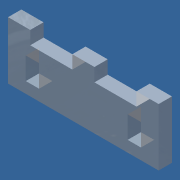
# Autodesk Inventor part: link2p1press
Saved by Autodesk Inventor 2014 (Build 180170000, 170)
## iProperties
Created: 2013-09-11
Part Number: link2p1press
Material: Glass
Document SubType Name: Modeling
Designer: Lefo
Density: 2.18 g/cm^3
Appearance: Clear
Author: Lefo
Autodesk Inventor part; units mm, degrees
ref_plane "YZ Plane" through (0, 0, 0) normal (1, 0, 0) x (0, 1, 0)
ref_plane "XZ Plane" through (0, 0, 0) normal (0, 1, 0) x (-1, 0, 0)
ref_plane "XY Plane" through (0, 0, 0) normal (0, 0, 1) x (1, 0, 0)
sketch "Sketch1" plane through (0, 0, 0) normal (0, 1, 0) x (-1, 0, 0)
  line L0 (0, 0) -> (34, 0)
  line L1 (34, 0) -> (34, 3)
  line L2 (34, 3) -> (0, 3)
  line L3 (0, 3) -> (0, 0)
  dimension "d0" = 34
  dimension "d1" = 3
  constraints: 8 end point, 2 parallel, 1 horizontal, 1 perpendicular
  measures "d0" distance of L2.end L1.end
  measures "d1" distance of L1.end L0.end
extrude "Extrusion1" add sketch "Sketch1" along normal blind 10
sketch "Sketch2" plane through (0, 10, 0) normal (0, 1, 0) x (1, 0, 0)
  line L0 (-34, -3) -> (0, -3) projected
  line L1 (-34, 0) -> (-29, 0)
  line L2 (-29, 0) -> (-29, -3)
  line L3 (-29, -3) -> (-34, -3)
  line L4 (-34, -3) -> (-34, 0)
  line L5 (-5, 0) -> (0, 0)
  line L6 (0, 0) -> (0, -3)
  line L7 (0, -3) -> (-5, -3)
  line L8 (-5, -3) -> (-5, 0)
  line L9 (-19.5, 0) -> (-14.5, 0)
  line L10 (-14.5, 0) -> (-14.5, -3)
  line L11 (-14.5, -3) -> (-19.5, -3)
  line L12 (-19.5, -3) -> (-19.5, 0)
  dimension "d4" = 3
  dimension "d5" = 5
  dimension "d6" = 3
  dimension "d7" = 5
  dimension "d8" = 3
  dimension "d9" = 5
  dimension "d10" = 9.5
  constraints: 24 end point, 6 parallel, 3 horizontal, 3 perpendicular, 1 point on line
  measures "d4" distance of L1.end L2.end
  measures "d5" distance of L1.start L1.end
  measures "d6" distance of L0.end L5.end
  measures "d7" distance of L5.start L5.end
  measures "d8" distance of L10.end L9.end
  measures "d9" distance of L9.start L9.end
  measures "d10" distance between parallel lines of L8 L10
extrude "Extrusion2" add sketch "Sketch2" along normal blind 3
sketch "Sketch4" plane through (0, 0, 0) normal (0, 0, -1) x (-1, 0, 0)
  line L0 (34, 0) -> (34, 13) projected
  line L1 (30, 2.5) -> (27, 2.5)
  line L2 (27, 2.5) -> (27, 7.5)
  line L3 (27, 7.5) -> (30, 7.5)
  line L4 (30, 7.5) -> (30, 2.5)
  line L5 (0, 0) -> (34, 0) projected
  line L6 (0, 0) -> (0, 13) projected
  line L7 (17, 0) -> (17, 25.0309) construction
  line L8 (7, 2.5) -> (7, 7.5)
  line L9 (4, 2.5) -> (7, 2.5)
  line L10 (7, 7.5) -> (4, 7.5)
  line L11 (4, 7.5) -> (4, 2.5)
  line L12 (19.5, 10) -> (29, 10) projected
  dimension "d17" = 3
  dimension "d18" = 5
  dimension "d22" = 2.5
  dimension "d23" = 4
  dimension "d25" = 10
  constraints: 18 end point, 4 symmetric about line, 3 parallel, 1 horizontal, 1 midpoint, 1 perpendicular
  measures "d17" distance of L2.end L3.end
  measures "d18" distance of L2.start L2.end
  measures "d22" distance between parallel lines of L5 L1
  measures "d23" distance between parallel lines of L0 L4
  measures "d25" distance between parallel lines of L5 L12
extrude "Extrusion4" cut sketch "Sketch4" against normal blind 3
equation "\"d22\" = -0.5 * d18 + 0.5 * d25"
body "Solid1"
